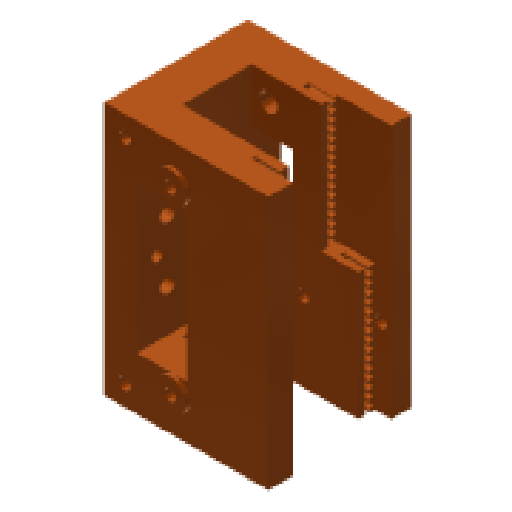
# Autodesk Inventor part: Toolhead Base
Saved by Autodesk Inventor 2023.2 (Build 272271000, 271)
## iProperties
Created: 2023-02-04
Part Number: Toolhead Base
Material: ABS Plastic
Document SubType Name: Modeling
Designer: remop
Density: 1.06 g/cm^3
Appearance: Smooth - Light Orange
Author: remop
Autodesk Inventor part; units mm, degrees
ref_plane "YZ Plane" through (0, 0, 0) normal (1, 0, 0) x (0, 1, 0)
ref_plane "XZ Plane" through (0, 0, 0) normal (0, 1, 0) x (-1, 0, 0)
ref_plane "XY Plane" through (0, 0, 0) normal (0, 0, 1) x (1, 0, 0)
sketch "Sketch1" plane through (0, 0, 0) normal (0, 0, 1) x (1, 0, 0)
  circle A0 centre (42.2396, 26.5) radius 2.25 projected
  circle A1 centre (42.2396, -23.5) radius 2.25 projected
  circle A2 centre (42.2396, -23.5) radius 6
  circle A3 centre (42.2396, 26.5) radius 6
  line L0 (48.2396, -23.5) -> (48.2396, -16.5)
  line L1 (48.2396, -16.5) -> (34.2396, -16.5)
  line L2 (34.2396, -16.5) -> (28.2396, -22.5)
  line L3 (28.2396, -22.5) -> (28.2396, -29.5)
  line L4 (28.2396, -29.5) -> (42.2396, -29.5)
  line L5 (48.2396, 26.5) -> (48.2396, 19.5)
  line L6 (48.2396, 19.5) -> (28.2396, 19.5)
  line L7 (28.2396, 19.5) -> (28.2396, 32.5)
  line L8 (28.2396, 32.5) -> (42.2396, 32.5)
  line L9 (42.2396, -29.5) -> (48.2396, -29.5)
  line L10 (48.2396, -29.5) -> (48.2396, -23.5)
  line L11 (48.2396, 26.5) -> (48.2396, 32.5)
  line L12 (48.2396, 32.5) -> (42.2396, 32.5)
  point P0 (0, 0)
  dimension "d0" = 12
  dimension "d3" = 14
  dimension "d4" = 45
  dimension "d5" = 7
  dimension "d6" = 7
  constraints: 26 end point, 8 tangent, 5 perpendicular, 5 point on circle, 3 horizontal, 2 centre point, 2 coincident, 2 point on line, 2 vertical, 1 collinear, 1 equal radius, 1 parallel, 1 vertical alignment
  measures "d0" diameter of A2
  measures "d3" distance of L3.end L4.end
  measures "d4" angle of L2 L3
  measures "d5" distance of L0.start L0.end
  measures "d6" distance of L2.end L3.end
extrude "Extrusion1" add sketch "Sketch1" along normal blind 9
sketch "Sketch2" plane through (0, 0, 9) normal (0, 0, 1) x (1, 0, 0)
  line L0 (28.2396, 32.5) -> (28.2396, 19.5) projected
  line L1 (28.2396, 19.5) -> (48.2396, 19.5) projected
  line L2 (48.2396, 19.5) -> (48.2396, 32.5) projected
  circle A0 centre (42.2396, 26.5) radius 2.25 projected
  line L3 (48.2396, -16.5) -> (34.2396, -16.5) projected
  line L4 (34.2396, -16.5) -> (28.2396, -22.5) projected
  line L5 (28.2396, -22.5) -> (28.2396, -29.5) projected
  line L6 (28.2396, -29.5) -> (48.2396, -29.5) projected
  circle A1 centre (42.2396, -23.5) radius 2.25 projected
  line L7 (36.2396, -15.705) -> (36.2396, 18.995) projected
  line L8 (36.2396, -15.705) -> (46.2396, -15.705) projected
  line L9 (46.2396, 18.995) -> (46.2396, -15.705) projected
  line L10 (36.2396, 18.995) -> (46.2396, 18.995) projected
  line L11 (34.2396, -16.5) -> (28.2396, -22.5) projected
  line L12 (28.2396, 19.5) -> (28.2396, -22.5)
  line L13 (36.2396, -15.705) -> (36.2396, -16.5)
  line L14 (36.2396, 18.995) -> (36.2396, 19.5)
  line L15 (28.2396, 19.5) -> (48.2396, 19.5) projected
  line L16 (38.2396, 19.5) -> (38.2396, 32.5)
  line L17 (48.2396, -16.5) -> (34.2396, -16.5) projected
  line L18 (38.2396, -16.5) -> (38.2396, -29.5)
  line L19 (28.2396, -29.5) -> (42.2396, -29.5) projected
  circle A2 centre (20.2396, -6.5) radius 14 projected
  circle A3 centre (20.2396, -6.5) radius 15
  line L20 (48.2396, -29.5) -> (48.2396, -16.5) projected
  line L21 (48.2396, 32.5) -> (28.2396, 32.5) projected
  point P0 (0, 0)
  point P1 (38.2396, 19.5)
  point P2 (35.2396, -6.5)
  point P3 (28.2396, -19.1886)
  point P4 (28.2396, 6.1886)
  dimension "d7" = 1
  constraints: 10 end point, 6 point on line, 2 midpoint, 1 centre point, 1 coincident, 1 collinear, 1 perpendicular, 1 vertical, 1 vertical alignment
  measures "d7" radial gap between concentric circles of A2 A3
extrude "Extrusion2" add sketch "Sketch2" along normal blind 10 contours L21 L16 L1 L0 | L1 L14 L7 L13 L3 L4 L12 A3 | L4 L3 L18 L6 L5
sketch "Sketch3" plane through (0, 0, 19) normal (0, 0, 1) x (1, 0, 0)
  line L0 (28.2396, -29.5) -> (38.2396, -29.5) projected
  line L1 (38.2396, -29.5) -> (38.2396, -16.5) projected
  line L2 (38.2396, -16.5) -> (36.2396, -16.5) projected
  line L3 (36.2396, -16.5) -> (36.2396, 19.5) projected
  line L4 (36.2396, 19.5) -> (38.2396, 19.5) projected
  line L5 (28.2396, 32.5) -> (28.2396, 6.1886) projected
  arc A0 (28.2396, -19.1886) -> (28.2396, 6.1886) centre (20.2396, -6.5) ccw projected
  line L6 (28.2396, -19.1886) -> (28.2396, -29.5) projected
  line L7 (28.2396, 19.5) -> (28.2396, 6.1886) projected
  line L8 (28.2396, -19.1886) -> (28.2396, -22.5) projected
  line L9 (28.2396, 6.1886) -> (28.2396, -19.1886)
  line L10 (38.2396, 32.5) -> (28.2396, 32.5) projected
  line L11 (38.2396, 19.5) -> (38.2396, 32.5) projected
  point P0 (0, 0)
  constraints: 2 end point, 1 vertical
extrude "Extrusion3" add sketch "Sketch3" along normal blind 12 contours L6 A0 L5 L10 L11 L4 L3 L2 L1 L0
sketch "Sketch5" plane through (0, 0, 9) normal (0, 0, -1) x (-1, 0, 0)
  line L0 (-28.2396, 19.5) -> (-36.2396, 19.5) projected
  line L1 (-36.2396, -16.5) -> (-36.2396, 19.5) projected
  line L2 (-36.2396, -16.5) -> (-34.2396, -16.5) projected
  line L3 (-34.2396, -16.5) -> (-28.2396, -22.5) projected
  line L4 (-28.2396, -19.1886) -> (-28.2396, -22.5) projected
  arc A0 (-28.2396, 6.1886) -> (-28.2396, -19.1886) centre (-20.2396, -6.5) ccw projected
  line L5 (-28.2396, 19.5) -> (-28.2396, 6.1886) projected
  arc A1 (-28.2396, 6.1886) -> (-28.2396, -19.1886) centre (-20.2396, -6.5) ccw projected
  line L6 (-31.2396, 3.698) -> (-36.2396, 3.698)
  line L7 (-36.2396, -16.5) -> (-36.2396, 19.5) projected
  point P0 (0, 0)
  dimension "d12" = 5
  constraints: 2 end point, 1 perpendicular, 1 point on circle, 1 point on line
  measures "d12" distance of L6.start L6.end
extrude "Extrusion4" add sketch "Sketch5" along normal up to surface (9 mm away) contours L5 A0 L6 L1 L0
sketch "Sketch7" plane through (0, 0, 31) normal (0, 0, 1) x (1, 0, 0)
  line L0 (28.2396, 32.5) -> (28.2396, 6.1886) projected
  arc A0 (28.2396, -19.1886) -> (28.2396, 6.1886) centre (20.2396, -6.5) ccw projected
  line L1 (28.2396, -19.1886) -> (28.2396, -29.5) projected
  line L2 (28.2396, -29.5) -> (38.2396, -29.5) projected
  line L3 (38.2396, -29.5) -> (38.2396, -16.5) projected
  line L4 (38.2396, -16.5) -> (36.2396, -16.5) projected
  line L5 (36.2396, -16.5) -> (36.2396, 19.5) projected
  line L6 (36.2396, 19.5) -> (38.2396, 19.5) projected
  line L7 (38.2396, 19.5) -> (38.2396, 32.5) projected
  line L8 (38.2396, 32.5) -> (28.2396, 32.5) projected
  arc A1 (31.2396, 3.698) -> (28.2396, 6.1886) centre (20.2396, -6.5) ccw projected
  line L9 (28.2396, -19.1886) -> (28.2396, 6.1886)
  point P0 (0, 0)
  constraints: 2 end point, 1 vertical
extrude "Extrusion5" add sketch "Sketch7" against normal blind 10 contours A0 L9
sketch "Sketch6" plane through (28.2396, 6.1886, 0) normal (-1, 0, 0) x (0, 0, 1)
  circle A0 centre (27.5, 2.9564) radius 1.2295 projected
  line L0 (0, 26.3114) -> (0, 0) projected
  line L1 (0, 0) -> (21, 0) projected
  line L2 (31, 26.3114) -> (31, -35.6886) projected
  line L3 (0, 26.3114) -> (31, 26.3114) projected
  circle A1 centre (7.5, 2.9564) radius 1.2295 projected
  circle A2 centre (27.5, -12.0436) radius 1.2295 projected
  circle A3 centre (7.5, -12.0436) radius 1.2295 projected
  line L4 (0, -28.6886) -> (0, -35.6886) projected
  line L5 (0, -35.6886) -> (31, -35.6886) projected
  line L6 (21, -25.3772) -> (21, 0) projected
  line L7 (9, -25.3772) -> (21, -25.3772) projected
  line L8 (9, -25.3772) -> (9, -28.6886) projected
  line L9 (0, -28.6886) -> (9, -28.6886) projected
  point P0 (0, -6.1886)
hole "Hole1" at (28.2396, -5.855, 27.5) at (28.2396, 9.145, 27.5) at (28.2396, 9.145, 7.5) direction (1, 0, 0) diameter 3.6 end through all counterbore diameter 6.5 counterbore depth 3.4 clearance for "Socket Head Cap Screw ISO 4762" size "M3" standard "ISO"
sketch "Sketch8" plane through (38.2396, -29.5, 9) normal (1, 0, 0) x (0, 0, -1)
  line L0 (0, 13) -> (0, 0) projected
  line L1 (0, 13) -> (-22, 13) projected
  line L2 (-22, 0) -> (-22, 13) projected
  line L3 (0, 0) -> (-22, 0) projected
  line L4 (0, 62) -> (0, 49) projected
  line L5 (0, 62) -> (-22, 62) projected
  line L6 (-22, 49) -> (-22, 62) projected
  line L7 (0, 49) -> (-22, 49) projected
  line L8 (-22, 49) -> (9, 49) projected
  line L9 (-26, 62) -> (-17, 62)
  line L10 (-17, 62) -> (-17, 49)
  line L11 (-17, 49) -> (-26, 49)
  line L12 (-26, 49) -> (-26, 62)
  line L13 (0, 13) -> (-22, 13) projected
  line L14 (-26, 0) -> (-17, 0)
  line L15 (-17, 0) -> (-17, 13)
  line L16 (-17, 13) -> (-26, 13)
  line L17 (-26, 13) -> (-26, 0)
  point P0 (9, 29.5)
  point P1 (-17, 49)
  point P2 (-17, 0)
  point P3 (-17, 13)
  dimension "d24" = 17
  dimension "d25" = 4
  constraints: 16 end point, 4 parallel, 3 point on line, 2 horizontal, 2 perpendicular, 1 vertical alignment
  measures "d24" distance between parallel lines of L15 L0
  measures "d25" distance between parallel lines of L17 L2
extrude "Extrusion6" add sketch "Sketch8" along normal up to surface (10 mm away) contours L15 L3 L2 L1 | L2 L14 L17 L16 | L10 L7 L6 L5 | L6 L11 L12 L9
sketch "Sketch9" plane through (0, 0, 31) normal (0, 0, 1) x (1, 0, 0)
  line L0 (28.2396, 32.5) -> (28.2396, -29.5) projected
  line L1 (28.2396, -29.5) -> (38.2396, -29.5) projected
  line L2 (38.2396, -29.5) -> (38.2396, -16.5) projected
  line L3 (38.2396, -16.5) -> (36.2396, -16.5) projected
  line L4 (36.2396, -16.5) -> (36.2396, 19.5) projected
  line L5 (36.2396, 19.5) -> (38.2396, 19.5) projected
  line L6 (38.2396, 19.5) -> (38.2396, 32.5) projected
  line L7 (38.2396, 32.5) -> (28.2396, 32.5) projected
  point P0 (0, 0)
extrude "Extrusion7" add sketch "Sketch9" along normal up to surface (4 mm away)
sketch "Sketch10" plane through (48.2396, 19.5, 26) normal (1, 0, 0) x (0, 0, -1)
  line L0 (0, 13) -> (0, 0) projected
  line L1 (-9, 13) -> (0, 13) projected
  line L2 (-9, 0) -> (-9, 13) projected
  line L3 (0, 0) -> (-9, 0) projected
  line L4 (-9, -49) -> (-9, -36) projected
  line L5 (0, -49) -> (-9, -49) projected
  line L6 (0, -36) -> (0, -49) projected
  line L7 (-9, -36) -> (0, -36) projected
  line L8 (26, -49) -> (26, -36) projected
  line L9 (26, -36) -> (17, -36) projected
  line L10 (17, -49) -> (17, -36) projected
  line L11 (26, -49) -> (17, -49) projected
  line L12 (26, 0) -> (26, 13) projected
  line L13 (26, 13) -> (17, 13) projected
  line L14 (17, 0) -> (17, 13) projected
  line L15 (26, 0) -> (17, 0) projected
  line L16 (26, 0) -> (26, -15.802) projected
  line L17 (26, 0) -> (26, -36)
  line L18 (17, -36) -> (17, -15.802) projected
  line L19 (17, -36) -> (17, 0)
  line L20 (0, 13) -> (0, 0) projected
  line L21 (0, 0) -> (0, -36)
  line L22 (17, -36) -> (-9, -36) projected
  line L23 (-9, -36) -> (-9, 0)
  point P0 (26, -19.5)
  constraints: 8 end point, 3 collinear, 1 perpendicular
extrude "Extrusion8" add sketch "Sketch10" along normal blind 1
sketch "Sketch11" plane through (49.2396, 19.5, 26) normal (1, 0, 0) x (0, 0, -1)
  line L0 (0, -49) -> (0, 13) projected
  line L1 (0, 13) -> (-9, 13) projected
  line L2 (-9, 13) -> (-9, -49) projected
  line L3 (-9, -49) -> (0, -49) projected
  line L4 (26, -49) -> (26, 13) projected
  line L5 (26, 13) -> (17, 13) projected
  line L6 (17, 13) -> (17, -49) projected
  line L7 (17, -49) -> (26, -49) projected
  line L8 (17, 13) -> (17, -49) projected
  line L9 (26, -36) -> (26, 0) projected
  line L10 (26, -18) -> (17, -18)
  line L11 (0, -49) -> (0, 13) projected
  line L12 (0, -18) -> (-9, -18)
  line L13 (-9, 0) -> (-9, -36) projected
  point P0 (0, -18)
  constraints: 4 end point, 4 midpoint
extrude "Extrusion9" add sketch "Sketch11" along normal blind 9 contours L12 L2 L1 L0 | L7 L6 L10 L4
sketch "Sketch12" plane through (49.2396, 19.5, 26) normal (1, 0, 0) x (0, 0, -1)
  line L0 (17, -18) -> (26, -18) projected
  line L1 (26, -18) -> (26, 13) projected
  line L2 (26, 13) -> (17, 13) projected
  line L3 (17, 13) -> (17, -18) projected
  line L4 (0, -18) -> (-9, -18) projected
  line L5 (-9, -18) -> (-9, -49) projected
  line L6 (-9, -49) -> (0, -49) projected
  line L7 (0, -49) -> (0, -18) projected
  line L8 (-3, -23) -> (-3, -163.2) projected
  line L9 (18.5, -13) -> (18.5, -18)
  line L10 (17, -18) -> (26, -18) projected
  line L11 (-3, -23) -> (-3, -18)
  line L12 (0, -18) -> (-9, -18) projected
  arc A0 (-1.5, -48) -> (-1.5, -47) centre (-1.5, -47.5) ccw
  arc A1 (-1.5, -48) -> (-1.5, -49) centre (-1.5, -48.5) ccw
  line L13 (-9, -49) -> (0, -49) projected
  line L14 (-1.5, -47) -> (-1.5, -49) construction
  line L15 (26, -49) -> (-9, -49) projected
  arc A2 (-1.5, -46) -> (-1.5, -45) centre (-1.5, -45.5) ccw
  arc A3 (-1.5, -46) -> (-1.5, -47) centre (-1.5, -46.5) ccw
  arc A4 (-1.5, -44) -> (-1.5, -43) centre (-1.5, -43.5) ccw
  arc A5 (-1.5, -44) -> (-1.5, -45) centre (-1.5, -44.5) ccw
  arc A6 (-1.5, -42) -> (-1.5, -41) centre (-1.5, -41.5) ccw
  arc A7 (-1.5, -42) -> (-1.5, -43) centre (-1.5, -42.5) ccw
  arc A8 (-1.5, -40) -> (-1.5, -39) centre (-1.5, -39.5) ccw
  arc A9 (-1.5, -40) -> (-1.5, -41) centre (-1.5, -40.5) ccw
  arc A10 (-1.5, -38) -> (-1.5, -37) centre (-1.5, -37.5) ccw
  arc A11 (-1.5, -38) -> (-1.5, -39) centre (-1.5, -38.5) ccw
  arc A12 (-1.5, -36) -> (-1.5, -35) centre (-1.5, -35.5) ccw
  arc A13 (-1.5, -36) -> (-1.5, -37) centre (-1.5, -36.5) ccw
  arc A14 (-1.5, -34) -> (-1.5, -33) centre (-1.5, -33.5) ccw
  arc A15 (-1.5, -34) -> (-1.5, -35) centre (-1.5, -34.5) ccw
  arc A16 (-1.5, -32) -> (-1.5, -31) centre (-1.5, -31.5) ccw
  arc A17 (-1.5, -32) -> (-1.5, -33) centre (-1.5, -32.5) ccw
  arc A18 (-1.5, -30) -> (-1.5, -29) centre (-1.5, -29.5) ccw
  arc A19 (-1.5, -30) -> (-1.5, -31) centre (-1.5, -30.5) ccw
  arc A20 (-1.5, -28) -> (-1.5, -27) centre (-1.5, -27.5) ccw
  arc A21 (-1.5, -28) -> (-1.5, -29) centre (-1.5, -28.5) ccw
  arc A22 (-1.5, -26) -> (-1.5, -25) centre (-1.5, -25.5) ccw
  arc A23 (-1.5, -26) -> (-1.5, -27) centre (-1.5, -26.5) ccw
  arc A24 (-1.5, -24) -> (-1.5, -23) centre (-1.5, -23.5) ccw
  arc A25 (-1.5, -24) -> (-1.5, -25) centre (-1.5, -24.5) ccw
  arc A26 (-1.5, -22) -> (-1.5, -21) centre (-1.5, -21.5) ccw
  arc A27 (-1.5, -22) -> (-1.5, -23) centre (-1.5, -22.5) ccw
  arc A28 (-1.5, -20) -> (-1.5, -19) centre (-1.5, -19.5) ccw
  arc A29 (-1.5, -20) -> (-1.5, -21) centre (-1.5, -20.5) ccw
  arc A30 (-1.5, -18) -> (-1.5, -17) centre (-1.5, -17.5) ccw
  arc A31 (-1.5, -18) -> (-1.5, -19) centre (-1.5, -18.5) ccw
  arc A32 (-1.5, -16) -> (-1.5, -15) centre (-1.5, -15.5) ccw
  arc A33 (-1.5, -16) -> (-1.5, -17) centre (-1.5, -16.5) ccw
  arc A34 (-1.5, -14) -> (-1.5, -13) centre (-1.5, -13.5) ccw
  arc A35 (-1.5, -14) -> (-1.5, -15) centre (-1.5, -14.5) ccw
  arc A36 (-1.5, -12) -> (-1.5, -11) centre (-1.5, -11.5) ccw
  arc A37 (-1.5, -12) -> (-1.5, -13) centre (-1.5, -12.5) ccw
  arc A38 (-1.5, -10) -> (-1.5, -9) centre (-1.5, -9.5) ccw
  arc A39 (-1.5, -10) -> (-1.5, -11) centre (-1.5, -10.5) ccw
  arc A40 (20, 12) -> (20, 13) centre (20, 12.5) ccw
  arc A41 (20, 12) -> (20, 11) centre (20, 11.5) ccw
  line L16 (26, 13) -> (-9, 13) projected
  line L17 (20, 13) -> (20, 11) construction
  line L18 (18.5, 127.2) -> (18.5, -13) projected
  arc A42 (20, 10) -> (20, 9) centre (20, 9.5) ccw
  arc A43 (20, 10) -> (20, 11) centre (20, 10.5) ccw
  arc A44 (20, 8) -> (20, 7) centre (20, 7.5) ccw
  arc A45 (20, 8) -> (20, 9) centre (20, 8.5) ccw
  arc A46 (20, 6) -> (20, 5) centre (20, 5.5) ccw
  arc A47 (20, 6) -> (20, 7) centre (20, 6.5) ccw
  arc A48 (20, 4) -> (20, 3) centre (20, 3.5) ccw
  arc A49 (20, 4) -> (20, 5) centre (20, 4.5) ccw
  arc A50 (20, 2) -> (20, 1) centre (20, 1.5) ccw
  arc A51 (20, 2) -> (20, 3) centre (20, 2.5) ccw
  arc A52 (20, 0) -> (20, -1) centre (20, -0.5) ccw
  arc A53 (20, 0) -> (20, 1) centre (20, 0.5) ccw
  arc A54 (20, -2) -> (20, -3) centre (20, -2.5) ccw
  arc A55 (20, -2) -> (20, -1) centre (20, -1.5) ccw
  arc A56 (20, -4) -> (20, -5) centre (20, -4.5) ccw
  arc A57 (20, -4) -> (20, -3) centre (20, -3.5) ccw
  arc A58 (20, -6) -> (20, -7) centre (20, -6.5) ccw
  arc A59 (20, -6) -> (20, -5) centre (20, -5.5) ccw
  arc A60 (20, -8) -> (20, -9) centre (20, -8.5) ccw
  arc A61 (20, -8) -> (20, -7) centre (20, -7.5) ccw
  arc A62 (20, -10) -> (20, -11) centre (20, -10.5) ccw
  arc A63 (20, -10) -> (20, -9) centre (20, -9.5) ccw
  arc A64 (20, -12) -> (20, -13) centre (20, -12.5) ccw
  arc A65 (20, -12) -> (20, -11) centre (20, -11.5) ccw
  arc A66 (20, -14) -> (20, -15) centre (20, -14.5) ccw
  arc A67 (20, -14) -> (20, -13) centre (20, -13.5) ccw
  arc A68 (20, -16) -> (20, -17) centre (20, -16.5) ccw
  arc A69 (20, -16) -> (20, -15) centre (20, -15.5) ccw
  arc A70 (20, -18) -> (20, -19) centre (20, -18.5) ccw
  arc A71 (20, -18) -> (20, -17) centre (20, -17.5) ccw
  point P0 (26, -19.5)
  point P1 (20, 13)
  point P2 (-3, -49)
  point P3 (-1.5, -47)
  point P4 (-1.5, -49)
  point P5 (-1.5, -18)
  point P6 (-1.5, -19)
  point P7 (-1.5, -21)
  point P8 (-1.5, -23)
  point P9 (-1.5, -25)
  point P10 (-1.5, -27)
  point P11 (-1.5, -29)
  point P12 (-1.5, -31)
  point P13 (-1.5, -33)
  point P14 (-1.5, -35)
  point P15 (-1.5, -37)
  point P16 (-1.5, -39)
  point P17 (-1.5, -41)
  point P18 (-1.5, -43)
  point P19 (-1.5, -45)
  point P20 (18.5, 13)
  point P21 (20, 11)
  point P22 (20, 9)
  point P23 (20, 7)
  point P24 (20, 5)
  point P25 (20, 3)
  point P26 (20, 1)
  point P27 (20, -11)
  point P28 (20, -13)
  point P29 (20, -15)
  point P30 (20, -17)
  dimension "d35" = 1
  dimension "d36" = 1.5
  dimension "d39" = 2
  dimension "d94" = 1.5
  dimension "d97" = 2
  constraints: 144 point on circle, 72 centre point, 8 end point, 4 point on line, 4 tangent, 3 equal radius, 2 midpoint, 2 perpendicular, 2 vertical, 2 vertical alignment, 1 coincident, 1 parallel, 238 other
  measures "d35" distance of A1.centre A0.centre
  measures "d36" distance from line of L8 A1.centre
  measures "d39" distance of A0.centre A2.centre
  measures "d94" distance from line of L18 A40.centre
  measures "d97" distance of A41.centre A42.centre
extrude "Belts_Bottom" add sketch "Sketch12" along normal blind 6 contours L3 L2 L18 L9 L0 | A71 A68 A69 A66 A67 A64 A65 A62 A63 A60 A61 A58 A59 A56 A57 A54 A55 A52 A53 A50 A51 A48 A49 A46 A47 A44 A45 A42 A43 A41 A40 L2 L1 L0 | L7 L6 A1 A0 A3 A2 A5 A4 A7 A6 A9 A8 A11 A10 A13 A12 A15 A14 A17 A16 A19 A18 A21 A20 A23 A22 A25 A24 A27 A26 A29 A28 A31 L4 | L11 L8 L6 L5 L4
sketch "Sketch13" plane through (58.2396, 19.5, 26) normal (1, 0, 0) x (0, 0, -1)
  line L0 (-3, -13) -> (-3, 127.2) projected
  line L1 (-9, 13) -> (-9, -18) projected
  line L2 (-9, -18) -> (0, -18) projected
  line L3 (0, -18) -> (0, 13) projected
  line L4 (0, 13) -> (-9, 13) projected
  line L5 (26, -49) -> (26, -18) projected
  line L6 (26, -18) -> (17, -18) projected
  line L7 (17, -18) -> (17, -49) projected
  line L8 (17, -49) -> (26, -49) projected
  line L9 (-9, -18) -> (-3, -18) projected
  line L10 (-3, -13) -> (-3, -18)
  arc A0 (20, -48) -> (20, -49) centre (20, -48.5) ccw
  line L11 (17, -49) -> (26, -49) projected
  arc A1 (20, -48) -> (20, -47) centre (20, -47.5) ccw
  line L12 (20, -49) -> (20, -47) construction
  arc A2 (-1.5, 13) -> (-1.5, 12) centre (-1.5, 12.5) ccw
  line L13 (26, 13) -> (-9, 13) projected
  arc A3 (-1.5, 11) -> (-1.5, 12) centre (-1.5, 11.5) ccw
  line L14 (-1.5, 13) -> (-1.5, 11) construction
  arc A4 (-1.5, 9) -> (-1.5, 10) centre (-1.5, 9.5) ccw
  arc A5 (-1.5, 11) -> (-1.5, 10) centre (-1.5, 10.5) ccw
  arc A6 (-1.5, 7) -> (-1.5, 8) centre (-1.5, 7.5) ccw
  arc A7 (-1.5, 9) -> (-1.5, 8) centre (-1.5, 8.5) ccw
  arc A8 (-1.5, 5) -> (-1.5, 6) centre (-1.5, 5.5) ccw
  arc A9 (-1.5, 7) -> (-1.5, 6) centre (-1.5, 6.5) ccw
  arc A10 (-1.5, 3) -> (-1.5, 4) centre (-1.5, 3.5) ccw
  arc A11 (-1.5, 5) -> (-1.5, 4) centre (-1.5, 4.5) ccw
  arc A12 (-1.5, 1) -> (-1.5, 2) centre (-1.5, 1.5) ccw
  arc A13 (-1.5, 3) -> (-1.5, 2) centre (-1.5, 2.5) ccw
  arc A14 (-1.5, -1) -> (-1.5, 0) centre (-1.5, -0.5) ccw
  arc A15 (-1.5, 1) -> (-1.5, 0) centre (-1.5, 0.5) ccw
  arc A16 (-1.5, -3) -> (-1.5, -2) centre (-1.5, -2.5) ccw
  arc A17 (-1.5, -1) -> (-1.5, -2) centre (-1.5, -1.5) ccw
  arc A18 (-1.5, -5) -> (-1.5, -4) centre (-1.5, -4.5) ccw
  arc A19 (-1.5, -3) -> (-1.5, -4) centre (-1.5, -3.5) ccw
  arc A20 (-1.5, -7) -> (-1.5, -6) centre (-1.5, -6.5) ccw
  arc A21 (-1.5, -5) -> (-1.5, -6) centre (-1.5, -5.5) ccw
  arc A22 (-1.5, -9) -> (-1.5, -8) centre (-1.5, -8.5) ccw
  arc A23 (-1.5, -7) -> (-1.5, -8) centre (-1.5, -7.5) ccw
  arc A24 (-1.5, -11) -> (-1.5, -10) centre (-1.5, -10.5) ccw
  arc A25 (-1.5, -9) -> (-1.5, -10) centre (-1.5, -9.5) ccw
  arc A26 (-1.5, -13) -> (-1.5, -12) centre (-1.5, -12.5) ccw
  arc A27 (-1.5, -11) -> (-1.5, -12) centre (-1.5, -11.5) ccw
  arc A28 (-1.5, -15) -> (-1.5, -14) centre (-1.5, -14.5) ccw
  arc A29 (-1.5, -13) -> (-1.5, -14) centre (-1.5, -13.5) ccw
  arc A30 (-1.5, -17) -> (-1.5, -16) centre (-1.5, -16.5) ccw
  arc A31 (-1.5, -15) -> (-1.5, -16) centre (-1.5, -15.5) ccw
  arc A32 (-1.5, -19) -> (-1.5, -18) centre (-1.5, -18.5) ccw
  arc A33 (-1.5, -17) -> (-1.5, -18) centre (-1.5, -17.5) ccw
  line L15 (18.5, -163.2) -> (18.5, -23) projected
  line L16 (18.5, -23) -> (18.5, -18)
  arc A34 (20, -46) -> (20, -45) centre (20, -45.5) ccw
  arc A35 (20, -46) -> (20, -47) centre (20, -46.5) ccw
  arc A36 (20, -44) -> (20, -43) centre (20, -43.5) ccw
  arc A37 (20, -44) -> (20, -45) centre (20, -44.5) ccw
  arc A38 (20, -42) -> (20, -41) centre (20, -41.5) ccw
  arc A39 (20, -42) -> (20, -43) centre (20, -42.5) ccw
  arc A40 (20, -40) -> (20, -39) centre (20, -39.5) ccw
  arc A41 (20, -40) -> (20, -41) centre (20, -40.5) ccw
  arc A42 (20, -38) -> (20, -37) centre (20, -37.5) ccw
  arc A43 (20, -38) -> (20, -39) centre (20, -38.5) ccw
  arc A44 (20, -36) -> (20, -35) centre (20, -35.5) ccw
  arc A45 (20, -36) -> (20, -37) centre (20, -36.5) ccw
  arc A46 (20, -34) -> (20, -33) centre (20, -33.5) ccw
  arc A47 (20, -34) -> (20, -35) centre (20, -34.5) ccw
  arc A48 (20, -32) -> (20, -31) centre (20, -31.5) ccw
  arc A49 (20, -32) -> (20, -33) centre (20, -32.5) ccw
  arc A50 (20, -30) -> (20, -29) centre (20, -29.5) ccw
  arc A51 (20, -30) -> (20, -31) centre (20, -30.5) ccw
  arc A52 (20, -28) -> (20, -27) centre (20, -27.5) ccw
  arc A53 (20, -28) -> (20, -29) centre (20, -28.5) ccw
  arc A54 (20, -26) -> (20, -25) centre (20, -25.5) ccw
  arc A55 (20, -26) -> (20, -27) centre (20, -26.5) ccw
  arc A56 (20, -24) -> (20, -23) centre (20, -23.5) ccw
  arc A57 (20, -24) -> (20, -25) centre (20, -24.5) ccw
  arc A58 (20, -22) -> (20, -21) centre (20, -21.5) ccw
  arc A59 (20, -22) -> (20, -23) centre (20, -22.5) ccw
  arc A60 (20, -20) -> (20, -19) centre (20, -19.5) ccw
  arc A61 (20, -20) -> (20, -21) centre (20, -20.5) ccw
  arc A62 (20, -18) -> (20, -17) centre (20, -17.5) ccw
  arc A63 (20, -18) -> (20, -19) centre (20, -18.5) ccw
  point P0 (26, -19.5)
  point P1 (-3, 13)
  point P2 (-1.5, 11)
  point P3 (-1.5, 9)
  point P4 (-1.5, 7)
  point P5 (-1.5, 5)
  point P6 (-1.5, 3)
  point P7 (-1.5, 1)
  point P8 (-1.5, -1)
  point P9 (-1.5, -3)
  point P10 (-1.5, -5)
  point P11 (-1.5, -7)
  point P12 (-1.5, -9)
  point P13 (-1.5, -11)
  point P14 (-1.5, -13)
  point P15 (-1.5, -15)
  point P16 (-1.5, -18)
  point P17 (20, -18)
  point P18 (20, -19)
  point P19 (20, -21)
  point P20 (20, -23)
  point P21 (20, -25)
  point P22 (20, -27)
  point P23 (20, -29)
  point P24 (20, -31)
  point P25 (20, -33)
  point P26 (20, -35)
  point P27 (20, -37)
  point P28 (20, -39)
  point P29 (20, -41)
  point P30 (20, -43)
  point P31 (20, -45)
  point P32 (20, -47)
  point P33 (18.5, -49)
  dimension "d54" = 1
  dimension "d63" = 1.5
  dimension "d66" = 2
  dimension "d88" = 2
  dimension "d93" = 1.5
  constraints: 128 point on circle, 64 centre point, 8 end point, 4 tangent, 3 equal radius, 3 point on line, 3 vertical, 2 midpoint, 2 perpendicular, 2 vertical alignment, 210 other
  measures "d54" diameter of A0
  measures "d63" distance from line of L0 A2.centre
  measures "d66" distance of A3.centre A4.centre
  measures "d88" distance of A1.centre A34.centre
  measures "d93" distance from line of L15 A43.centre
extrude "Belts_Top" add sketch "Sketch13" along normal blind 6 contours L10 L2 L1 L4 L0 | L4 L3 L2 A33 A30 A31 A28 A29 A26 A27 A24 A25 A22 A23 A20 A21 A18 A19 A16 A17 A14 A15 A12 A13 A10 A11 A8 A9 A6 A7 A4 A5 A3 A2 | L8 A0 A1 A35 A34 A37 A36 A39 A38 A41 A40 A43 A42 A45 A44 A47 A46 A49 A48 A51 A50 A53 A52 A55 A54 A57 A56 A59 A58 A61 A60 A63 L6 L5 | L8 L7 L6 L16 L15
sketch "Sketch14" plane through (55.2396, 19.5, 26) normal (1, 0, 0) x (0, 0, -1)
  line L0 (-9, -49) -> (-3, -49) projected
  line L1 (-3, -49) -> (-3, -18) projected
  line L2 (-9, -18) -> (-3, -18) projected
  line L3 (-9, -18) -> (-9, -49) projected
  line L4 (26, 13) -> (20, 13) projected
  line L5 (18.5, -18) -> (17, -18) projected
  line L6 (26, -18) -> (26, 13) projected
  line L7 (18.5, 13) -> (17, 13) projected
  line L8 (17, 13) -> (17, -18) projected
  line L9 (18.5, -18) -> (18.5, 13) projected
  arc A0 (20, 12) -> (20, 13) centre (20, 12.5) ccw projected
  arc A1 (20, 12) -> (20, 11) centre (20, 11.5) ccw projected
  arc A2 (20, 10) -> (20, 11) centre (20, 10.5) ccw projected
  arc A3 (20, 10) -> (20, 9) centre (20, 9.5) ccw projected
  arc A4 (20, 8) -> (20, 9) centre (20, 8.5) ccw projected
  arc A5 (20, 8) -> (20, 7) centre (20, 7.5) ccw projected
  arc A6 (20, 6) -> (20, 7) centre (20, 6.5) ccw projected
  arc A7 (20, 6) -> (20, 5) centre (20, 5.5) ccw projected
  arc A8 (20, 4) -> (20, 5) centre (20, 4.5) ccw projected
  arc A9 (20, 4) -> (20, 3) centre (20, 3.5) ccw projected
  arc A10 (20, 2) -> (20, 3) centre (20, 2.5) ccw projected
  arc A11 (20, 2) -> (20, 1) centre (20, 1.5) ccw projected
  arc A12 (20, 0) -> (20, 1) centre (20, 0.5) ccw projected
  arc A13 (20, 0) -> (20, -1) centre (20, -0.5) ccw projected
  arc A14 (20, -2) -> (20, -1) centre (20, -1.5) ccw projected
  arc A15 (20, -2) -> (20, -3) centre (20, -2.5) ccw projected
  arc A16 (20, -4) -> (20, -3) centre (20, -3.5) ccw projected
  arc A17 (20, -4) -> (20, -5) centre (20, -4.5) ccw projected
  arc A18 (20, -6) -> (20, -5) centre (20, -5.5) ccw projected
  arc A19 (20, -6) -> (20, -7) centre (20, -6.5) ccw projected
  arc A20 (20, -8) -> (20, -7) centre (20, -7.5) ccw projected
  arc A21 (20, -8) -> (20, -9) centre (20, -8.5) ccw projected
  arc A22 (20, -10) -> (20, -9) centre (20, -9.5) ccw projected
  arc A23 (20, -10) -> (20, -11) centre (20, -10.5) ccw projected
  arc A24 (20, -12) -> (20, -11) centre (20, -11.5) ccw projected
  arc A25 (20, -12) -> (20, -13) centre (20, -12.5) ccw projected
  arc A26 (20, -14) -> (20, -13) centre (20, -13.5) ccw projected
  arc A27 (20, -14) -> (20, -15) centre (20, -14.5) ccw projected
  arc A28 (20, -16) -> (20, -15) centre (20, -15.5) ccw projected
  arc A29 (20, -16) -> (20, -17) centre (20, -16.5) ccw projected
  arc A30 (20, -18) -> (20, -17) centre (20, -17.5) ccw projected
  line L10 (26, -18) -> (20, -18) projected
  line L11 (26, -18) -> (20, -18) projected
  line L12 (21, -18) -> (21, 13)
  line L13 (26, 13) -> (-9, 13) projected
  point P0 (26, -19.5)
  point P1 (21, 13)
  dimension "d102" = 5
  constraints: 2 end point, 2 point on line, 1 perpendicular
  measures "d102" distance between parallel lines of L6 L12
extrude "Walls" add sketch "Sketch14" along normal up to surface (9 mm away) contours L3 L2 L1 L0 | L6 L10 L12 L4
sketch "Sketch18" plane through (28.2396, -29.5, 35) normal (0, 0, 1) x (1, 0, 0)
  line L0 (8, 13) -> (20, 13) projected
  line L1 (8, 49) -> (8, 13) projected
  line L2 (8, 49) -> (20, 49) projected
  line L3 (20, 49) -> (20, 13) projected
  line L4 (0, 0) -> (36, 0) projected
  line L5 (36, 62) -> (36, 0) projected
  line L6 (0, 62) -> (36, 62) projected
  line L7 (0, 0) -> (0, 62) projected
  circle A0 centre (17, 52.92) radius 1.75 projected
  circle A1 centre (17, 9.08) radius 1.75 projected
  circle A2 centre (17, 52.92) radius 3.92
  circle A3 centre (17, 9.08) radius 3.92
  circle A4 centre (17, 52.92) radius 1.4
  circle A5 centre (17, 9.08) radius 1.4
  point P0 (-28.2396, 29.5)
  dimension "d111" = 2.8
  constraints: 4 centre point, 4 coincident, 2 tangent, 1 equal radius
  measures "d111" diameter of A4
extrude "Extrusion15" add sketch "Sketch18" along normal blind 1 contours A2 | A3 | A0 | A1
sketch "Sketch19" plane through (28.2396, -29.5, 0) normal (-1, 0, 0) x (0, 0, 1)
  arc A0 (8.8498, 35.6886) -> (6.1502, 35.6886) centre (7.5, 38.645) ccw projected
  line L0 (8.8498, 35.6886) -> (21, 35.6886) projected
  line L1 (21, 10.3114) -> (21, 35.6886) projected
  line L2 (9, 10.3114) -> (21, 10.3114) projected
  line L3 (9, 10.3114) -> (9, 7) projected
  line L4 (0, 7) -> (9, 7) projected
  line L5 (0, 7) -> (0, 0) projected
  line L6 (0, 0) -> (35, 0) projected
  line L7 (35, 0) -> (35, 62) projected
  line L8 (0, 62) -> (35, 62) projected
  line L9 (0, 62) -> (0, 35.6886) projected
  line L10 (0, 35.6886) -> (6.1502, 35.6886) projected
  circle A1 centre (27.5, 23.645) radius 3.25 projected
  circle A2 centre (27.5, 38.645) radius 3.25 projected
  point P0 (0, 29.5)
  point P1 (5.0002, 52)
  point P2 (20, 52.0744)
  dimension "d112" = 15
  dimension "d113" = 20
  dimension "d114" = 10
  measures "d112" distance of point (20, 52.074) point (5, 52)
  measures "d113" distance from line of L9 point (20, 52.074)
  measures "d114" distance from line of point (5, 52) L8
hole "Hole2" at (28.2396, 22.5, 5.0002) at (28.2396, 22.5744, 20) direction (1, 0, 0) diameter 2.8 depth 9
sketch "Sketch20" plane through (28.2396, -29.5, 0) normal (-1, 0, 0) x (0, 0, 1)
  circle A0 centre (5.0002, 52) radius 1.4 projected
  circle A1 centre (20, 52.0744) radius 1.4 projected
  arc A2 (8.8498, 35.6886) -> (6.1502, 35.6886) centre (7.5, 38.645) ccw projected
  line L0 (8.8498, 35.6886) -> (21, 35.6886) projected
  line L1 (21, 10.3114) -> (21, 35.6886) projected
  line L2 (9, 10.3114) -> (21, 10.3114) projected
  line L3 (9, 10.3114) -> (9, 7) projected
  line L4 (0, 7) -> (9, 7) projected
  line L5 (0, 7) -> (0, 0) projected
  line L6 (0, 0) -> (35, 0) projected
  line L7 (35, 0) -> (35, 62) projected
  line L8 (0, 62) -> (35, 62) projected
  line L9 (0, 62) -> (0, 35.6886) projected
  line L10 (0, 35.6886) -> (6.1502, 35.6886) projected
  circle A3 centre (27.5, 23.645) radius 3.25 projected
  circle A4 centre (27.5, 38.645) radius 3.25 projected
  point P0 (0, 29.5)
  point P1 (30, 11.145)
  point P2 (30, 31.145)
  dimension "d122" = 15
  dimension "d123" = 7.5
  dimension "d124" = 5
  dimension "d125" = 20
  constraints: 1 vertical alignment
  measures "d122" distance of A4.centre A3.centre
  measures "d123" vertical distance of A3.centre point (30, 31.145)
  measures "d124" distance from line of L7 point (30, 31.145)
  measures "d125" distance of point (30, 11.145) point (30, 31.145)
hole "Hole3" at (28.2396, -18.355, 30) at (28.2396, 1.645, 30) direction (1, 0, 0) diameter 2.8 depth 8 tip angle 118
sketch "Sketch21" plane through (64.2396, 19.5, 26) normal (1, 0, 0) x (0, 0, -1)
  line L0 (21, -18) -> (20, -18) projected
  arc A0 (20, -18) -> (20, -19) centre (20, -18.5) ccw projected
  arc A1 (20, -20) -> (20, -19) centre (20, -19.5) ccw projected
  arc A2 (20, -20) -> (20, -21) centre (20, -20.5) ccw projected
  arc A3 (20, -22) -> (20, -21) centre (20, -21.5) ccw projected
  arc A4 (20, -22) -> (20, -23) centre (20, -22.5) ccw projected
  arc A5 (20, -24) -> (20, -23) centre (20, -23.5) ccw projected
  arc A6 (20, -24) -> (20, -25) centre (20, -24.5) ccw projected
  arc A7 (20, -26) -> (20, -25) centre (20, -25.5) ccw projected
  arc A8 (20, -26) -> (20, -27) centre (20, -26.5) ccw projected
  arc A9 (20, -28) -> (20, -27) centre (20, -27.5) ccw projected
  arc A10 (20, -28) -> (20, -29) centre (20, -28.5) ccw projected
  arc A11 (20, -30) -> (20, -29) centre (20, -29.5) ccw projected
  arc A12 (20, -30) -> (20, -31) centre (20, -30.5) ccw projected
  arc A13 (20, -32) -> (20, -31) centre (20, -31.5) ccw projected
  arc A14 (20, -32) -> (20, -33) centre (20, -32.5) ccw projected
  arc A15 (20, -34) -> (20, -33) centre (20, -33.5) ccw projected
  arc A16 (20, -34) -> (20, -35) centre (20, -34.5) ccw projected
  arc A17 (20, -36) -> (20, -35) centre (20, -35.5) ccw projected
  arc A18 (20, -36) -> (20, -37) centre (20, -36.5) ccw projected
  arc A19 (20, -38) -> (20, -37) centre (20, -37.5) ccw projected
  arc A20 (20, -38) -> (20, -39) centre (20, -38.5) ccw projected
  arc A21 (20, -40) -> (20, -39) centre (20, -39.5) ccw projected
  arc A22 (20, -40) -> (20, -41) centre (20, -40.5) ccw projected
  arc A23 (20, -42) -> (20, -41) centre (20, -41.5) ccw projected
  arc A24 (20, -42) -> (20, -43) centre (20, -42.5) ccw projected
  arc A25 (20, -44) -> (20, -43) centre (20, -43.5) ccw projected
  arc A26 (20, -44) -> (20, -45) centre (20, -44.5) ccw projected
  arc A27 (20, -46) -> (20, -45) centre (20, -45.5) ccw projected
  arc A28 (20, -46) -> (20, -47) centre (20, -46.5) ccw projected
  arc A29 (20, -48) -> (20, -47) centre (20, -47.5) ccw projected
  arc A30 (20, -48) -> (20, -49) centre (20, -48.5) ccw projected
  line L1 (20, -49) -> (26, -49) projected
  line L2 (26, -49) -> (26, 13) projected
  line L3 (21, 13) -> (26, 13) projected
  line L4 (21, -18) -> (21, 13) projected
  line L5 (-3, 13) -> (-3, -49) projected
  line L6 (-3, 13) -> (-9, 13) projected
  line L7 (-9, 13) -> (-9, -49) projected
  line L8 (-3, -49) -> (-9, -49) projected
  line L9 (21, -18) -> (21, 13) projected
  line L10 (21, -18) -> (21, -49)
  line L11 (26, -49) -> (-9, -49) projected
  point P0 (26, -19.5)
  point P1 (21, -49)
  constraints: 2 end point, 1 perpendicular, 1 point on line
extrude "Extrusion16" add sketch "Sketch21" along normal blind 4 contours L4 L3 L2 L1 L10 | L5 L8 L7 L6
sketch "Sketch22" plane through (0, 0, 0) normal (0, 0, -1) x (-1, 0, 0)
  circle A0 centre (-65.7396, -10.2) radius 1.5 projected
  circle A1 centre (-50.7396, -10.2) radius 1.5 projected
  point P0 (0, 0)
hole "Hole4" at (65.7396, -10.2, 0) at (50.7396, -10.2, 0) direction (0, 0, 1) diameter 2.7 depth 10 tip angle 118
sketch "Sketch23" plane through (28.2396, -29.5, 35) normal (0, 0, 1) x (1, 0, 0)
  line L0 (0, 62) -> (40, 62) projected
  circle A0 centre (17, 9.08) radius 1.75 projected
  circle A1 centre (17, 52.92) radius 1.75 projected
  line L1 (0, 0) -> (0, 62) projected
  line L2 (0, 0) -> (40, 0) projected
  point P0 (-28.2396, 29.5)
  point P1 (5, 57)
  point P2 (5, 5)
  dimension "d142" = 5
  dimension "d143" = 5
  dimension "d144" = 5
  constraints: 1 vertical alignment
  measures "d142" distance from line of L1 point (5, 5)
  measures "d143" distance from line of L2 point (5, 5)
  measures "d144" distance from line of L0 point (5, 57)
hole "Hole5" at (33.2396, 27.5, 35) at (33.2396, -24.5, 35) at (45.2396, 23.42, 35) at (45.2396, -20.42, 35) direction (0, 0, -1) diameter 2.8 depth 9 tip angle 118
equation "\"d63\" = d55"
equation "\"d144\" = d143"
equation "\"d55\" = 1.5"
body "Solid1"
